Autodesk Fusion 360 part; units mm, degrees
note: some values were not read from the file. Chosen so that the rebuilt part matches the saved one: which bodies a step acts on.
(part 3 of 3)
equation "d601 = print_wall_t * 5"
equation "d605 = lip_h"
equation "d607 = lip_h"
equation "d639 = base_t * 6"
equation "d641 = base_t * 6"
equation "d643 = base_t * 6"
equation "d645 = base_t * 6"
equation "d657 = side_t * 6"
equation "d659 = side_t * 6"
equation "m2_clear_d = 2.2 mm" comment "M2 clearance hole for small electronics module mounting"
equation "roll_pin_d = 2 mm" comment "Roll pin diameter through shaft+bar - shock-resistant weapon fastening, stronger than friction set-screw alone"
equation "d693 = spinner_bar_W * 3"
equation "d695 = spinner_bar_W * 3"
named bodies: "Base_Plate_Al", "Left_Side_Plate_Al", "Right_Side_Plate_Al", "Left_Wheel", "Right_Wheel", "Top_Cover", "TT_Gearbox_L", "TT_Motor_Can_L", "TT_Gearbox_R", "TT_Motor_Can_R", "Battery_and_Tray", "Hammer_Servo", "Hammer_Arm", "Hammer_Head", "Front_Wedge_L", "Front_Wedge_R", "Spinner_Shaft", "Left_Support", "Right_Support", "Spinner_Sweep_Envelope", "Spinner_Motor", "Spinner_Bar", "Standoff_1", "Standoff_2", "Standoff_3", "Standoff_4", "Battery_Holder", "Spinner_Motor_Cradle", "TT_Motor_Mount_L", "TT_Motor_Clamp_L", "TT_Motor_Mount_R", "TT_Motor_Clamp_R", "Batt_Post_1", "Batt_Post_2", "Batt_Post_3", "Batt_Post_4", "Disconnect_Post_1", "Disconnect_Post_2", "Rear_Panel", "Weapon_Pulley", "Motor_Pulley", "ESC_Tekko32", "Holder_ESC_Tekko32", "Rx_ER6", "Holder_Rx_ER6", "UBEC_5A", "Holder_UBEC_5A", "DRV8874_A", "Holder_DRV8874_A", "DRV8874_B", "Holder_DRV8874_B", "ESP32_DevKit", "ESP32_Module", "ESP32_Dupont_Keepout_A", "ESP32_Dupont_Keepout_B", "Holder_ESP32", "FingerTech_Switch_Adapter", "FingerTech_Mini_Switch_Envelope"
